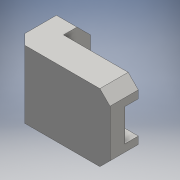
# Autodesk Inventor part: 240503_3Dsketch10
Saved by Autodesk Inventor 2016 (Build 200138000, 138)
## iProperties
Created: 2024-05-03
Part Number: 240503_3Dsketch10
Material: 일반
Document SubType Name: Modeling
Designer: pc
Density: 1 g/cm^3
Appearance: 기본값
Author: pc
Autodesk Inventor part; units mm, degrees
ref_plane "YZ Plane" through (0, 0, 0) normal (1, 0, 0) x (0, 1, 0)
ref_plane "XZ Plane" through (0, 0, 0) normal (0, 1, 0) x (-1, 0, 0)
ref_plane "XY Plane" through (0, 0, 0) normal (0, 0, 1) x (1, 0, 0)
sketch "스케치1" plane through (0, 0, 0) normal (0, 0, 1) x (1, 0, 0)
  line L0 (14.1048, -8.184) -> (-14.1048, -8.184)
  line L1 (-14.1048, -8.184) -> (-14.1048, 8.184)
  line L2 (-14.1048, 8.184) -> (14.1048, 8.184)
  line L3 (14.1048, 8.184) -> (14.1048, -8.184)
  line L4 (14.1048, -8.184) -> (-14.1048, 8.184) construction
  line L5 (-14.1048, -8.184) -> (14.1048, 8.184) construction
  point P0 (0, 0)
  constraints: 12 end point, 2 midpoint, 2 parallel, 1 horizontal, 1 perpendicular
extrude "돌출1" add sketch "스케치1" along normal blind 20
sketch "스케치2" plane through (-14.1048, 8.184, 0) normal (0, 1, 0) x (1, 0, 0)
  line L0 (0, -20) -> (28.2096, -20) projected
  line L1 (28.2096, 0) -> (0, 0) projected
  line L2 (6.0629, -20) -> (28.2096, -20)
  line L3 (28.2096, -20) -> (28.2096, 0)
  line L4 (28.2096, 0) -> (6.0629, 0)
  line L5 (6.0629, 0) -> (6.0629, -20)
  point P0 (14.1048, 0)
  constraints: 8 end point, 2 parallel, 1 horizontal, 1 perpendicular, 1 point on line
extrude "돌출2" cut sketch "스케치2" against normal blind 8
sketch "스케치3" plane through (-14.1048, 0.184, 0) normal (0, 1, 0) x (1, 0, 0)
  line L0 (6.0629, -20) -> (6.0629, 0) projected
  line L1 (28.2096, 0) -> (28.2096, -20) projected
  line L2 (6.0629, -5.1676) -> (28.2096, -5.1676)
  line L3 (28.2096, -5.1676) -> (28.2096, -14.7078)
  line L4 (28.2096, -14.7078) -> (6.0629, -14.7078)
  line L5 (6.0629, -14.7078) -> (6.0629, -5.1676)
  point P0 (14.1048, 0)
  constraints: 8 end point, 2 parallel, 2 point on line, 1 horizontal, 1 perpendicular
extrude "돌출3" cut sketch "스케치3" against normal blind 4
sketch "스케치4" plane through (-8.0419, 8.184, 20) normal (1, 0, 0) x (0, 0, -1)
  point P0 (20, -8.184)
sketch "스케치5" plane through (-8.0419, 8.184, 20) normal (1, 0, 0) x (0, 0, -1)
  line L0 (5.2922, -8) -> (5.2922, -12) projected
  line L1 (5.2922, -12) -> (14.8018, -12)
  line L2 (14.8018, -12) -> (14.8018, -4.7287)
  line L3 (14.8018, -4.7287) -> (5.2922, -4.7287)
  line L4 (5.2922, -4.7287) -> (5.2922, -12)
  point P0 (20, -8.184)
  constraints: 8 end point, 2 parallel, 1 horizontal, 1 perpendicular
extrude "돌출4" cut sketch "스케치5" against normal blind 10
chamfer "모따기1" distance 4 angle 45 1 edges at (-11.0733, 8.184, 20)
chamfer "모따기2" distance 4 angle 45 1 edges at (-11.0733, 8.184, 0)
chamfer "모따기3" distance 3 angle 45 1 edges at (14.1048, -4, 20)
chamfer "모따기4" distance 3 angle 45 1 edges at (14.1048, -4, 0)
chamfer "모따기5" distance 3 angle 45 1 edges at (-14.1048, -8.184, 10)
